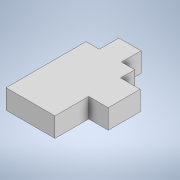
# Autodesk Inventor part: CotéV2
Saved by Autodesk Inventor 2020 (Build 240168000, 168)
## iProperties
Created: 2019-11-14
Part Number: CotéV2
Material: Générique
Document SubType Name: Modeling
Designer: erwan
Density: 1 g/cm^3
Appearance: Par défaut
Author: erwan
Autodesk Inventor part; units mm, degrees
ref_plane "YZ Plane" through (0, 0, 0) normal (1, 0, 0) x (0, 1, 0)
ref_plane "XZ Plane" through (0, 0, 0) normal (0, 1, 0) x (-1, 0, 0)
ref_plane "XY Plane" through (0, 0, 0) normal (0, 0, 1) x (1, 0, 0)
sketch "Esquisse1" plane through (0, 0, 0) normal (0, 1, 0) x (-1, 0, 0)
  line L0 (68.888, 27.0027) -> (13.888, 27.0027)
  line L1 (13.888, 27.0027) -> (13.888, -10.9973)
  line L2 (13.888, -62.9973) -> (28.888, -62.9973)
  line L3 (68.888, -62.9973) -> (68.888, 27.0027)
  line L4 (13.888, -10.9973) -> (-8.112, -10.9973)
  line L5 (-8.112, -10.9973) -> (-8.112, -46.9973)
  line L6 (-8.112, -46.9973) -> (13.888, -46.9973)
  line L7 (13.888, -46.9973) -> (13.888, -62.9973)
  line L8 (53.888, -62.9973) -> (53.888, -84.9973)
  line L9 (53.888, -84.9973) -> (28.888, -84.9973)
  line L10 (28.888, -84.9973) -> (28.888, -62.9973)
  line L11 (53.888, -62.9973) -> (68.888, -62.9973)
  point P0 (0, 0)
  dimension "d0" = 90
  dimension "d1" = 55
  dimension "d2" = 22
  dimension "d3" = 38
  dimension "d4" = 36
  dimension "d7" = 22
  dimension "d8" = 25
  dimension "d9" = 15
  dimension "d10" = 15
  constraints: 24 end point, 6 parallel, 3 perpendicular, 2 horizontal
  measures "d0" distance between parallel lines of L0 L2
  measures "d1" distance between parallel lines of L1 L3
  measures "d2" distance between parallel lines of L5 L1
  measures "d3" distance between parallel lines of L0 L4
  measures "d4" distance between parallel lines of L4 L6
  measures "d7" distance between parallel lines of L2 L9
  measures "d8" distance between parallel lines of L10 L8
  measures "d9" distance between parallel lines of L7 L10
  measures "d10" distance between parallel lines of L8 L3
extrude "Extrusion1" add sketch "Esquisse1" along normal blind 22
